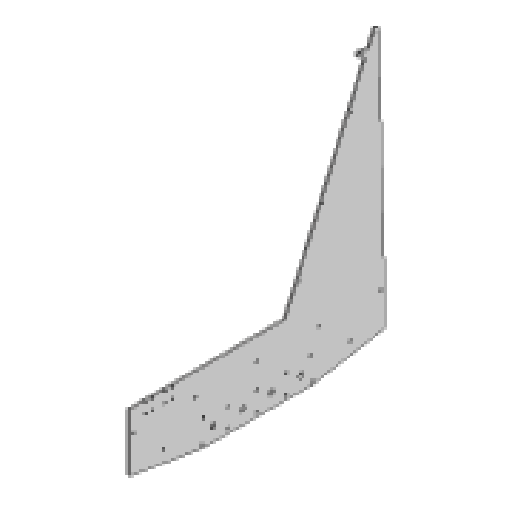
# Autodesk Inventor part: Outside Chassi Plate low 2.0
Saved by Autodesk Inventor 2023 (Build 270158000, 158)
## iProperties
Created: 2022-09-05
Part Number: Outside Chassi Plate low 2.0
Material: Generic
Document SubType Name: Modeling
Designer: deli
Density: 1 g/cm^3
Appearance: Default
Author: deli
Autodesk Inventor part; units mm, degrees
ref_plane "YZ Plane" through (0, 0, 0) normal (1, 0, 0) x (0, 1, 0)
ref_plane "XZ Plane" through (0, 0, 0) normal (0, 1, 0) x (-1, 0, 0)
ref_plane "XY Plane" through (0, 0, 0) normal (0, 0, 1) x (1, 0, 0)
sketch "Sketch1" plane through (0, 0, 0) normal (1, 0, 0) x (0, 1, 0)
  line L0 (-213.0456, 516.9078) -> (-298.6456, 516.9078)
  line L1 (-298.6456, 516.9078) -> (-316.9722, 411.201)
  line L2 (-213.0456, 139.2078) -> (-298.6456, 139.2078)
  circle A0 centre (-289.0456, 466.9078) radius 2
  circle A1 centre (-289.0456, 466.9078) radius 48 construction
  arc A2 (-277.1545, 465.8665) -> (-300.9116, 468.2046) centre (-289.0456, 466.9078) ccw construction
  circle A3 centre (-289.0456, 189.2078) radius 48 construction
  arc A4 (-300.9116, 187.911) -> (-277.1545, 190.2492) centre (-289.0456, 189.2078) ccw construction
  circle A5 centre (-289.0456, 189.2078) radius 2
  circle A6 centre (-296.2956, 393.2443) radius 4
  circle A7 centre (-296.2956, 262.8714) radius 4
  circle A8 centre (-296.2956, 393.2443) radius 18.75 construction
  circle A9 centre (-296.2956, 262.8714) radius 18.75 construction
  arc A10 (-308.9527, 394.6275) -> (-283.6118, 392.1334) centre (-296.2956, 393.2443) ccw construction
  arc A11 (-283.6118, 263.9822) -> (-308.9527, 261.4882) centre (-296.2956, 262.8714) ccw construction
  line L3 (-277.1545, 465.8665) -> (-283.6118, 392.1334) construction
  line L4 (-308.9527, 394.6275) -> (-300.9116, 468.2046) construction
  line L5 (-283.6118, 263.9822) -> (-277.1545, 190.2492) construction
  line L6 (-300.9116, 187.911) -> (-308.9527, 261.4882) construction
  circle A12 centre (-282.6598, 284.7146) radius 2
  circle A13 centre (-309.9315, 284.7146) radius 2
  circle A14 centre (-312.0456, 245.7688) radius 2
  circle A15 centre (-278.2187, 248.25) radius 2
  circle A16 centre (-246.0456, 511.9078) radius 2
  arc A17 (-317.0456, 229.9036) -> (-317.0456, 229.9036) centre (-294.2956, 229.9036) ccw
  line L7 (-317.0456, 245.7688) -> (-317.0456, 229.9036)
  arc A18 (-316.9722, 411.201) -> (-317.0456, 410.3469) centre (-312.0456, 410.3469) ccw
  line L8 (-317.0456, 410.3469) -> (-317.0456, 229.9036)
  line L9 (-298.6456, 139.2078) -> (-316.9722, 244.9147)
  circle A19 centre (-278.2187, 407.8657) radius 2
  arc A20 (-317.0456, 245.7688) -> (-316.9722, 244.9147) centre (-312.0456, 245.7688) ccw
  circle A21 centre (-246.0456, 236.1328) radius 2
  line L10 (-213.0456, 516.9078) -> (-213.0456, 285.8158)
  circle A22 centre (-246.0456, 419.9828) radius 2
  circle A23 centre (-246.0456, 328.0578) radius 2
  circle A24 centre (-312.0456, 410.3469) radius 2
  circle A25 centre (-246.0456, 144.2078) radius 2
  line L11 (-179.3811, 271.3598) -> (-182.1431, 264.9277)
  line L12 (-182.1431, 264.9277) -> (93.5164, 146.556)
  line L13 (93.5164, 146.556) -> (96.2784, 152.9881)
  line L14 (628.6384, -183.2052) -> (619.1262, -197.2948) construction
  line L15 (-182.3379, 277.146) -> (-189.0456, 261.5253) construction
  line L16 (-188.4024, 279.7501) -> (108.5747, 152.2244) construction
  line L17 (102.5102, 154.8285) -> (95.8025, 139.2078) construction
  line L18 (95.8025, 139.2078) -> (-189.0456, 261.5253) construction
  line L19 (-184.6634, 284.4023) -> (-173.6371, 279.6674) construction
  line L20 (-173.6371, 279.6674) -> (-175.2154, 275.992) construction
  line L21 (-175.2154, 275.992) -> (-186.2417, 280.7268) construction
  line L22 (-186.2417, 280.7268) -> (-184.6634, 284.4023) construction
  line L23 (-185.4431, 286.6416) -> (-176.0707, 282.617) construction
  line L24 (-178.4381, 277.1038) -> (-187.8106, 281.1284) construction
  line L25 (-176.0707, 282.617) -> (-176.6626, 281.2387) construction
  line L26 (-178.4381, 277.1038) -> (-179.03, 275.7255) construction
  line L27 (-176.6626, 281.2387) -> (-186.035, 285.2633) construction
  arc A26 (-185.4431, 286.6416) -> (-188.4024, 279.7501) centre (-186.9228, 283.1959) ccw construction
  arc A27 (-186.035, 285.2633) -> (-187.8106, 281.1284) centre (-186.9228, 283.1959) ccw construction
  line L28 (99.2023, 156.249) -> (99.7941, 157.6273) construction
  line L29 (99.7941, 157.6273) -> (109.1666, 153.6027) construction
  arc A28 (109.1666, 153.6027) -> (110.9421, 157.7376) centre (110.0544, 155.6701) ccw construction
  line L30 (110.9421, 157.7376) -> (101.5697, 161.7622) construction
  line L31 (101.5697, 161.7622) -> (102.1616, 163.1405) construction
  line L32 (102.1616, 163.1405) -> (111.534, 159.1158) construction
  arc A29 (108.5747, 152.2244) -> (111.534, 159.1158) centre (110.0544, 155.6701) ccw construction
  line L33 (109.3733, 158.1391) -> (107.795, 154.4637) construction
  line L34 (107.795, 154.4637) -> (96.7686, 159.1986) construction
  line L35 (96.7686, 159.1986) -> (98.3469, 162.874) construction
  line L36 (98.3469, 162.874) -> (109.3733, 158.1391) construction
  line L37 (93.5164, 146.556) -> (-213.0456, 139.2078)
  circle A30 centre (-173.8706, 265.1845) radius 1
  circle A31 centre (-91.1728, 229.673) radius 1
  circle A32 centre (5.3081, 188.2429) radius 1
  circle A33 centre (88.0059, 152.7314) radius 1
  circle A34 centre (73.8024, 176.6786) radius 1.5
  arc A35 (76.559, 175.4949) -> (71.0458, 177.8624) centre (73.8024, 176.6786) ccw
  line L38 (71.0458, 177.8624) -> (67.835, 170.3851)
  line L39 (76.559, 175.4949) -> (73.3482, 168.0176)
  line L40 (96.2784, 152.9881) -> (75.8451, 161.7624)
  line L41 (61.5798, 167.8881) -> (-213.0456, 285.8158)
  arc A36 (73.3482, 168.0176) -> (75.8451, 161.7624) centre (77.7243, 166.1385) ccw
  arc A37 (61.5798, 167.8881) -> (67.835, 170.3851) centre (63.4589, 172.2642) ccw
  circle A38 centre (73.8024, 176.6786) radius 6 construction
  circle A39 centre (-215.5456, 493.6078) radius 1.6
  circle A40 centre (-230.5456, 493.6078) radius 1.6
  circle A41 centre (-230.5456, 483.6078) radius 1.6
  circle A42 centre (-215.5456, 483.6078) radius 1.6
  circle A43 centre (-215.5456, 464.7078) radius 1.6
  circle A44 centre (-215.5456, 454.7078) radius 1.6
  circle A45 centre (-230.5456, 454.7078) radius 1.6
  circle A46 centre (-230.5456, 464.7078) radius 1.6
  line L42 (-215.5456, 493.6078) -> (-230.5456, 493.6078) construction
  line L43 (-230.5456, 493.6078) -> (-230.5456, 483.6078) construction
  line L44 (-230.5456, 483.6078) -> (-215.5456, 483.6078) construction
  line L45 (-215.5456, 483.6078) -> (-215.5456, 493.6078) construction
  line L46 (-215.5456, 454.7078) -> (-215.5456, 464.7078) construction
  line L47 (-215.5456, 464.7078) -> (-230.5456, 464.7078) construction
  line L48 (-230.5456, 464.7078) -> (-230.5456, 454.7078) construction
  line L49 (-230.5456, 454.7078) -> (-215.5456, 454.7078) construction
  line L50 (-296.2956, 393.2443) -> (-296.2956, 262.8714) construction
  circle A47 centre (-296.2956, 349.5578) radius 18.75 construction
  circle A48 centre (-296.2956, 306.5578) radius 18.75 construction
  line L51 (-241.0456, 516.9078) -> (-241.0456, 139.2078) construction
  circle A49 centre (-296.2956, 349.5578) radius 4
  circle A50 centre (-296.2956, 306.5578) radius 4
  circle A51 centre (-282.1248, 328.0578) radius 2
  circle A52 centre (-310.4665, 328.0578) radius 2
  circle A53 centre (-282.6598, 371.401) radius 2
  circle A54 centre (-309.9315, 371.401) radius 2
  point P0 (0, 0)
  point P1 (-317.0456, 245.7688)
  point P2 (-225.2933, 139.2078)
  dimension "d44" = 4
  dimension "d46" = 96
  dimension "d47" = 23.8732
  dimension "d51" = 23.8732
  dimension "d54" = 50
  dimension "d55" = 50
  dimension "d58" = 8
  dimension "d60" = 37.5
  dimension "d62" = 25.4648
  dimension "d64" = 178.768
  dimension "d65" = 178.768
  dimension "d66" = 178.768
  dimension "d67" = 178.768
  dimension "d68" = 74.0152
  dimension "d70" = 74.0152
  dimension "d94" = 2.5
  dimension "d95" = 2.5
  dimension "d103" = 4
  dimension "d124" = 28
  dimension "d142" = 4
  dimension "d143" = 2.5
  dimension "d144" = 4
  dimension "d145" = 4
  dimension "d146" = 18
  dimension "d147" = 18
  dimension "d148" = 5
  dimension "d149" = 5
  dimension "d153" = 4
  dimension "d218" = 0
  dimension "d235" = 33
  dimension "d244" = 28
  dimension "d246" = 85.5999
  dimension "d247" = 85.5999
  dimension "d258" = 5
  dimension "d259" = 5
  dimension "d260" = 4
  dimension "d261" = 4
  dimension "d266" = 33
  dimension "d267" = 33
  dimension "d268" = 91.925
  dimension "d269" = 91.925
  dimension "d270" = 91.925
  dimension "d277" = 5
  dimension "d296" = 33
  dimension "d297" = 7
  dimension "d317" = 0
  dimension "d333" = 377.7
  dimension "d334" = 5
  dimension "d336" = 17
  dimension "d338" = 5
  dimension "d339" = 5
  dimension "d340" = 300
  dimension "d342" = 4
  dimension "d343" = 12
  dimension "d344" = 7
  dimension "d345" = 6.6
  dimension "d346" = 2
  dimension "d347" = 10.2
  dimension "d348" = 1.5
  dimension "d349" = 1.5
  dimension "d350" = 3.75
  dimension "d351" = 1.5
  dimension "d353" = 3.75
  dimension "d354" = 6.6
  constraints: 104 end point, 55 centre point, 30 equal radius, 29 point on circle, 28 tangent, 24 perpendicular, 15 parallel, 13 coincident, 11 point on line, 5 vertical, 4 collinear, 4 concentric, 3 equal length
  measures "d44" diameter of A0
  measures "d46" diameter of A1
  measures "d47" diameter of A2
  measures "d51" diameter of A4
  measures "d54" distance from line of A0.centre L0
  measures "d55" distance from line of L2 A5.centre
  measures "d58" diameter of A6
  measures "d60" diameter of A8
  measures "d62" diameter of A10
  measures "d68" distance of L3.start L3.end
  measures "d70" distance of L5.start L5.end
  measures "d103" diameter of A16
  measures "d124" distance from line of A0.centre L7
  measures "d142" distance from line of L5 A15.centre
  measures "d144" distance from line of L3 A19.centre
  measures "d145" diameter of A19
  measures "d146" distance from line of A0.centre L1
  measures "d147" distance from line of L9 A3.centre
  measures "d148" radius of A18
  measures "d149" radius of A20
  measures "d153" diameter of A21
  measures "d218" horizontal distance of A0.centre A5.centre
  measures "d235" distance from line of L10 A16.centre
  measures "d244" distance edge to line of A1 L10
  measures "d246" distance of L2.start L2.end
  measures "d247" distance of L0.start L0.end
  measures "d260" diameter of A22
  measures "d261" diameter of A23
  measures "d266" distance from line of L10 A22.centre
  measures "d267" distance from line of L10 A23.centre
  measures "d268" distance of A22.centre A16.centre
  measures "d269" distance of A23.centre A22.centre
  measures "d270" distance of A21.centre A23.centre
  measures "d277" distance from line of L2 A25.centre
  measures "d296" distance from line of L10 A21.centre
  measures "d297" distance of L11.start L11.end
  measures "d317" horizontal distance of A25.centre A21.centre
  measures "d333" distance between parallel lines of L2 L0
  measures "d334" distance from line of L0 A16.centre
  measures "d336" distance between parallel lines of L18 L16
  measures "d338" distance between parallel lines of L11 L15
  measures "d339" distance between parallel lines of L13 L17
  measures "d340" distance of L11.end L12.end
  measures "d342" distance of L19.end L20.end
  measures "d343" distance of L19.start L19.end
  measures "d344" distance between parallel lines of L15 L20
  measures "d345" distance from line of L15 A26.centre
  measures "d346" distance from line of A26.centre L21
  measures "d347" distance of L23.start L23.end
  measures "d348" distance of L24.start L26.end
  measures "d349" distance of L23.end L25.end
  measures "d350" radius of A26
  measures "d351" distance of L28.start L28.end
  measures "d353" radius of A29
  measures "d354" distance from line of L17 A28.centre
extrude "Extrusion1" add sketch "Sketch1" along normal blind 3.175 contours L10 L41 L11 L12 L37 L2 L9 A17 A15 A14 A20 L8 A18 L1 L0 | L41 A37 L38 A35 L39 A36 L40 L13 L12 L11 | A17 A14 A15 L9
thread "Thread1" size "M2x0.4" class "6H" standard "ANSI Metric M Profile" full length
thread "Thread2" size "M2x0.4" class "6H" standard "ANSI Metric M Profile" full length
thread "Thread3" size "M2x0.4" class "6H" standard "ANSI Metric M Profile" full length
fillet "Fillet1" radius 2 2 edges at (1.5875, 96.2784, 152.9881) (1.5875, -213.0456, 285.8158)
thread "Thread4" size "M2x0.4" class "6H" standard "ANSI Metric M Profile" full length
body "Solid1"
